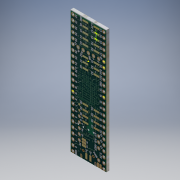
# Autodesk Inventor part: 101
Saved by Autodesk Inventor 2016 (Build 200138000, 138)
## iProperties
Created: 2014-04-22
Part Number: 101
Material: Plastica ABS
Document SubType Name: Modeling
Designer: larraguetajunior
Mass: 1.03972 g
Surface Area: 15.5511 cm^2
Volume: 0.980865 cm^3
Density: 1.06 g/cm^3
Appearance: Liscia - Bianco
Description: Teensy3.1 Board
GlobalPropertyList: <PropertyList/>
Author: larraguetajunior
Autodesk Inventor part; units mm, degrees
ref_plane "YZ Plane" through (0, 0, 0) normal (1, 0, 0) x (0, 1, 0)
ref_plane "XZ Plane" through (0, 0, 0) normal (0, 1, 0) x (-1, 0, 0)
ref_plane "XY Plane" through (0, 0, 0) normal (0, 0, 1) x (1, 0, 0)
sketch "Schizzo1" plane through (0, 0, 0) normal (0, 1, 0) x (-1, 0, 0)
  line L0 (-8.85, -43.18) -> (8.95, -43.18)
  line L1 (8.95, -43.18) -> (8.95, 17.78)
  line L2 (8.95, 17.78) -> (-8.85, 17.78)
  line L3 (-8.85, 17.78) -> (-8.85, -43.18)
  line L4 (-8.85, 17.78) -> (8.95, -43.18) construction
  line L5 (8.95, 17.78) -> (-8.85, -43.18) construction
  line L6 (8.95, 16.48) -> (-8.95, 16.48) construction
  line L7 (-7.6, 17.78) -> (-7.6, -43.18) construction
  circle A0 centre (-7.6, 16.48) radius 0.425
  circle A1 centre (-7.6, 13.94) radius 0.425
  circle A2 centre (-7.6, 11.4) radius 0.425
  circle A3 centre (-7.6, 8.86) radius 0.425
  circle A4 centre (-7.6, 6.32) radius 0.425
  circle A5 centre (-7.6, 3.78) radius 0.425
  circle A6 centre (-7.6, 1.24) radius 0.425
  circle A7 centre (-7.6, -1.3) radius 0.425
  circle A8 centre (-7.6, -3.84) radius 0.425
  circle A9 centre (-7.6, -6.38) radius 0.425
  circle A10 centre (-7.6, -8.92) radius 0.425
  circle A11 centre (-7.6, -11.46) radius 0.425
  circle A12 centre (-7.6, -14) radius 0.425
  circle A13 centre (-7.6, -16.54) radius 0.425
  circle A14 centre (-5.06, 16.48) radius 0.425
  circle A15 centre (-2.52, 16.48) radius 0.425
  circle A16 centre (0.02, 16.48) radius 0.425
  circle A17 centre (2.56, 16.48) radius 0.425
  circle A18 centre (5.1, 16.48) radius 0.425
  circle A19 centre (7.64, 16.48) radius 0.425
  circle A20 centre (7.64, 13.94) radius 0.425
  circle A21 centre (7.64, 11.4) radius 0.425
  circle A22 centre (7.64, 8.86) radius 0.425
  circle A23 centre (7.64, 6.32) radius 0.425
  circle A24 centre (7.64, 3.78) radius 0.425
  circle A25 centre (7.64, 1.24) radius 0.425
  circle A26 centre (7.64, -1.3) radius 0.425
  circle A27 centre (7.64, -3.84) radius 0.425
  circle A28 centre (7.64, -6.38) radius 0.425
  circle A29 centre (7.64, -8.92) radius 0.425
  circle A30 centre (7.64, -11.46) radius 0.425
  circle A31 centre (7.64, -14) radius 0.425
  circle A32 centre (7.64, -16.54) radius 0.425
  circle A33 centre (7.64, -19.08) radius 0.425
  circle A34 centre (7.64, -21.62) radius 0.425
  circle A35 centre (7.64, -24.16) radius 0.425
  circle A36 centre (7.64, -26.7) radius 0.425
  circle A37 centre (7.64, -29.24) radius 0.425
  circle A38 centre (7.64, -31.78) radius 0.425
  circle A39 centre (7.64, -34.32) radius 0.425
  circle A40 centre (7.64, -36.86) radius 0.425
  circle A41 centre (7.64, -39.4) radius 0.425
  circle A42 centre (7.64, -41.94) radius 0.425
  circle A43 centre (-7.6, -19.08) radius 0.425
  circle A44 centre (-7.6, -21.62) radius 0.425
  circle A45 centre (-7.6, -24.16) radius 0.425
  circle A46 centre (-7.6, -26.7) radius 0.425
  circle A47 centre (-7.6, -29.24) radius 0.425
  circle A48 centre (-7.6, -31.78) radius 0.425
  circle A49 centre (-7.6, -34.32) radius 0.425
  circle A50 centre (-7.6, -36.86) radius 0.425
  circle A51 centre (-7.6, -39.4) radius 0.425
  circle A52 centre (-7.6, -41.94) radius 0.425
  circle A53 centre (-5.06, -29.24) radius 0.425
  circle A54 centre (-2.52, -29.24) radius 0.425
  circle A55 centre (0.02, -29.24) radius 0.425
  circle A56 centre (2.56, -29.24) radius 0.425
  circle A57 centre (5.1, -29.24) radius 0.425
  point P0 (0, 0)
  point P1 (0.05, -12.7)
  dimension "d0" = 17.8
  dimension "d1" = 60.96
  dimension "d4" = 1.3
  dimension "d5" = 1.25
  dimension "d6" = 0.85
  dimension "d9" = 2.54
  dimension "d16" = 2.54
  dimension "d23" = 2.54
  dimension "d166" = 2.54
  dimension "d169" = 2.54
  constraints: 58 centre point, 16 end point, 4 point on line, 3 horizontal, 3 parallel, 2 midpoint, 2 perpendicular, 2 vertical, 112 other
  measures "d0" distance of L2.end L1.end
  measures "d1" distance of L1.end L0.end
  measures "d4" distance between parallel lines of L6 L2
  measures "d5" distance between parallel lines of L3 L7
  measures "d6" diameter of A0
  measures "d9" distance of A0.centre A1.centre
  measures "d16" distance of A0.centre A14.centre
  measures "d23" distance of A19.centre A20.centre
  measures "d166" distance of A47.centre A53.centre
  measures "d169" distance of A53.centre A54.centre
extrude "Estrusione2" add sketch "Schizzo1" along normal blind 1.6 contours L3 L2 L1 L0 | A14 | A15 | A16 | A17 | A18
fillet "Raccordo1" radius 0.2 12 edges at (-0.05, 0, 17.78) (-0.05, 1.6, 17.78) (8.85, 0.8, 17.78) (8.85, 0, -12.7) (8.85, 1.6, -12.7) (8.85, 0.8, -43.18) (-0.05, 0, -43.18) (-8.95, 0, -12.7) (-8.95, 0.8, -43.18) (-8.95, 0.8, 17.78) (-8.95, 1.6, -12.7) (-0.05, 1.6, -43.18)
ref_plane "Piano di lavoro1" through (0, 13.85, 0) normal (0, 1, 0) x (1, 0, 0)
sketch "Schizzo2" plane through (0, 13.85, 0) normal (0, 1, 0) x (1, 0, 0)
  line L0 (-8.9159, -19.3191) -> (-8.9159, 43.0633) construction
  line L1 (-8.9159, 43.0633) -> (8.8631, 43.0633) construction
  line L2 (8.8631, 43.0633) -> (8.8631, -19.3191) construction
  line L3 (8.8631, -19.3191) -> (-8.9159, -19.3191) construction
  constraints: 2 other
decal "Decalcomania1"
ref_plane "Piano di lavoro2" through (0, -10.75, 0) normal (0, -1, 0) x (1, 0, 0)
sketch "Schizzo3" plane through (0, -10.75, 0) normal (0, -1, 0) x (1, 0, 0)
  line L0 (9.0474, 17.6328) -> (9.0474, -44.6653) construction
  line L1 (9.0474, -44.6653) -> (-9.0191, -44.6653) construction
  line L2 (-9.0191, -44.6653) -> (-9.0191, 17.6328) construction
  line L3 (-9.0191, 17.6328) -> (9.0474, 17.6328) construction
  point P0 (0, 0)
  constraints: 2 other
decal "Decalcomania2"
sketch "Schizzo4" plane through (0, 1.6, 0) normal (0, 1, 0) x (1, 0, 0)
  circle A0 centre (7.6, 11.46) radius 0.425 projected
sketch "Schizzo5" plane through (0, 1.6, 0) normal (0, 1, 0) x (1, 0, 0)
  circle A0 centre (7.6, -1.24) radius 0.425 projected
sketch "Schizzo6" plane through (0, 1.6, 0) normal (0, 1, 0) x (1, 0, 0)
  circle A0 centre (7.6, -3.78) radius 0.425 projected
sketch "Schizzo7" plane through (0, 1.6, 0) normal (0, 1, 0) x (1, 0, 0)
  circle A0 centre (-7.64, 16.54) radius 0.425 projected
sketch "Schizzo8" plane through (0, 1.6, 0) normal (0, 1, 0) x (1, 0, 0)
  circle A0 centre (-7.64, 14) radius 0.425 projected
sketch "Schizzo9" plane through (0, 1.6, 0) normal (0, 1, 0) x (1, 0, 0)
  circle A0 centre (-7.64, 11.46) radius 0.425 projected
sketch "Sketch10" plane through (0, 0, 0) normal (0, -1, 0) x (1, 0, 0)
  circle A0 centre (7.6, -11.46) radius 0.425 projected
sketch "Schizzo11" plane through (0, 0, 0) normal (0, -1, 0) x (1, 0, 0)
  circle A0 centre (-7.64, -16.54) radius 0.425 projected
sketch "Schizzo12" plane through (0, 1.6, 0) normal (0, 1, 0) x (1, 0, 0)
  circle A0 centre (-7.64, -11.4) radius 0.425 projected
sketch "Schizzo13" plane through (0, 1.6, 0) normal (0, 1, 0) x (1, 0, 0)
  circle A0 centre (-7.64, -8.86) radius 0.425 projected
sketch "Schizzo14" plane through (0, 0, 0) normal (0, -1, 0) x (1, 0, 0)
  circle A0 centre (7.6, 1.24) radius 0.425 projected
sketch "Schizzo15" plane through (0, 0, 0) normal (0, -1, 0) x (1, 0, 0)
  circle A0 centre (7.6, 3.78) radius 0.425 projected
sketch "Sketch16" plane through (0, 0, 0) normal (0, -1, 0) x (1, 0, 0)
  point P0 (0, 0)
  point P1 (3.8313, 14.0194)
  point P2 (3.8313, 11.5063)
